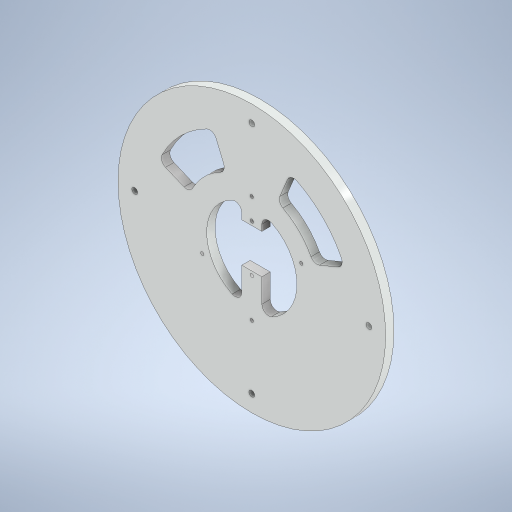
# Autodesk Inventor part: 아크릴 LED확산판
Saved by Autodesk Inventor 2023.1 (Build 271208000, 208)
## iProperties
Created: 2022-08-14
Part Number: 아크릴 LED확산판
Material: 일반
Document SubType Name: Modeling
Designer: fly01
Density: 1 g/cm^3
Appearance: 기본값
Author: fly01
Autodesk Inventor part; units mm, degrees
ref_plane "YZ Plane" through (0, 0, 0) normal (1, 0, 0) x (0, 1, 0)
ref_plane "XZ Plane" through (0, 0, 0) normal (0, 1, 0) x (-1, 0, 0)
ref_plane "XY Plane" through (0, 0, 0) normal (0, 0, 1) x (1, 0, 0)
sketch "스케치1" plane through (0, 0, 0) normal (0, 0, 1) x (1, 0, 0)
  circle A0 centre (0, 0) radius 80
  circle A1 centre (0, 0) radius 34 construction
  circle A2 centre (0, 0) radius 27
  circle A3 centre (0, 0) radius 60
  circle A4 centre (0, 0) radius 40
  line L0 (0, 0) -> (22.961, 55.4328)
  line L1 (0, 0) -> (55.4328, 22.961)
  line L2 (0, 0) -> (0, 60) construction
  point P0 (15.3073, 36.9552)
  point P1 (36.9552, 15.3073)
  dimension "d0" = 160
  dimension "d1" = 68
  dimension "d2" = 54
  dimension "d3" = 120
  dimension "d4" = 80
  dimension "d5" = 45
  dimension "d45" = 22.5
  constraints: 6 end point, 5 centre point, 5 coincident, 3 point on circle, 1 vertical
  measures "d0" diameter of A0
  measures "d1" diameter of A1
  measures "d2" diameter of A2
  measures "d3" diameter of A3
  measures "d4" diameter of A4
  measures "d5" angle of L0 L1
  measures "d45" angle of L2 L0
extrude "돌출1" add sketch "스케치1" along normal blind 5 contours A0 | A2 L1 A4 L0 | A2 L0 A4 L1 | L1 A3 L0 A4 | A4 L0 A3 L1
extrude "돌출2" cut sketch "스케치1" along normal blind 5 contours A4 L0 A3 L1 picked at (23.2061, 47.8488)
fillet "모깎기1" radius 4 4 edges at (22.961, 55.4328, 2.5) (15.3073, 36.9552, 2.5) (36.9552, 15.3073, 2.5) (55.4328, 22.961, 2.5)
sketch "스케치2" plane through (0, 0, 5) normal (0, 0, 1) x (1, 0, 0)
  circle A0 centre (0, 70) radius 1.75
  point P0 (0, 0)
  dimension "d14" = 3.5
  dimension "d15" = 70
  constraints: 1 centre point
  measures "d14" diameter of A0
  measures "d15" distance of point (0, 0) A0.centre
extrude "돌출3" cut sketch "스케치2" against normal blind 5
pattern_circular "원형 패턴2" count 4 over 360 about axis through (0, 0, 0) along (0, 0, 1) of "돌출3"
sketch "스케치3" plane through (0, 0, 5) normal (0, 0, 1) x (1, 0, 0)
  circle A0 centre (0, 0) radius 6 construction
  line L0 (-6, 16.5) -> (6, 16.5) construction
  line L1 (6, 16.5) -> (6, -6) construction
  line L2 (6, -6) -> (-6, -6) construction
  line L3 (-6, -6) -> (-6, 16.5) construction
  line L4 (-6, 21.35) -> (6, 21.35) construction
  line L5 (6, 21.35) -> (6, -10.85) construction
  line L6 (6, -10.85) -> (-6, -10.85) construction
  line L7 (-6, -10.85) -> (-6, 21.35) construction
  circle A1 centre (0, 19.35) radius 1.05
  line L8 (-6, 5.25) -> (-8.8851, 5.25) construction
  circle A2 centre (0, -8.85) radius 1.05
  line L9 (-6, 27) -> (6, 27)
  line L10 (6, 27) -> (6, 17)
  line L11 (6, 17) -> (-6, 17)
  line L12 (-6, 17) -> (-6, 27)
  line L13 (-6, -6.5) -> (6, -6.5)
  line L14 (6, -6.5) -> (6, -27)
  line L15 (6, -27) -> (-6, -27)
  line L16 (-6, -27) -> (-6, -6.5)
  circle A3 centre (0, 0) radius 27 projected
  point P0 (0, -6)
  point P1 (0, 27)
  point P2 (0, -27)
  point P3 (-6, -26.3249)
  point P4 (6, -26.3249)
  point P5 (6, 26.3249)
  point P6 (-6, 26.3249)
  dimension "d21" = 12
  dimension "d22" = 12
  dimension "d23" = 22.5
  dimension "d24" = 32.2
  dimension "d26" = 2.1
  dimension "d27" = 28.2
  dimension "d28" = 0.5
  dimension "d29" = 0.5
  dimension "d30" = 12
  dimension "d31" = 12
  constraints: 34 end point, 8 parallel, 5 horizontal, 5 midpoint, 4 perpendicular, 3 point on line, 2 centre point, 2 point on circle, 1 coincident, 1 symmetric about line, 1 vertical, 1 vertical alignment, 3 other
  measures "d22" distance of L0.start L0.end
  measures "d23" distance of L0.end L1.end
  measures "d24" distance of L6.end L4.start
  measures "d26" diameter of A1
  measures "d27" distance of A2.centre A1.centre
  measures "d28" distance between parallel lines of L0 L11
  measures "d29" distance between parallel lines of L2 L13
  measures "d30" distance of L9.start L9.end
  measures "d31" distance of L14.end L15.end
extrude "돌출4" add sketch "스케치3" against normal blind 5 contours A3 L10 L11 L12 | L16 L13 L14 A3
fillet "모깎기2" radius 4 4 edges at (-6, 26.3249, 2.5) (6, 26.3249, 2.5) (-6, -26.3249, 2.5) (6, -26.3249, 2.5)
sketch "스케치4" plane through (0, 0, 0) normal (0, 0, -1) x (-1, 0, 0)
  circle A0 centre (0, 0) radius 32.0565 construction
  circle A1 centre (0, -32.0565) radius 1
  line L0 (0, -32.0565) -> (0, 0)
  line L1 (0, 0) -> (29.6163, -12.2675)
  circle A2 centre (29.6163, -12.2675) radius 1
  circle A3 centre (0, 32.0565) radius 1
  circle A4 centre (-29.6163, 12.2675) radius 1
  dimension "d35" = 64.113
  dimension "d36" = 2
  dimension "d37" = 2
  dimension "d38" = 67.5
  dimension "d41" = 360
  constraints: 5 centre point, 4 end point, 2 coincident, 2 point on circle, 1 vertical, 9 other
  measures "d35" diameter of A0
  measures "d36" diameter of A1
  measures "d37" diameter of A2
  measures "d38" angle of L0 L1
extrude "돌출5" cut sketch "스케치4" against normal blind 5
mirror "미러1" about plane through (0, 0, 0) normal (1, 0, 0) of "돌출2", "모깎기1"
